Autodesk Fusion 360 part; units mm, degrees
note: some values were not read from the file. Set by a fixed rule: which sketch regions a step uses.
(part 43 of 59)
  spline S54 degree 5 poles (24.6806, -2.8132) (24.6807, -2.8132) (24.6809, -2.8133) (24.6812, -2.8135) (24.6816, -2.8138) (24.6822, -2.8142) (24.683, -2.8146) (24.6838, -2.8151) (24.6848, -2.8157) (24.6858, -2.8163) (24.6869, -2.8169) (24.6881, -2.8177) (24.6895, -2.8184) (24.6909, -2.8193) (24.6924, -2.8201) (24.694, -2.821) (24.6956, -2.822) (24.6974, -2.823) (24.6993, -2.8241) (24.7012, -2.8252) (24.7033, -2.8263) (24.7054, -2.8275) (24.7076, -2.8287) (24.7099, -2.83) (24.7122, -2.8313) (24.7147, -2.8327) (24.7172, -2.8341) (24.7198, -2.8355) (24.7225, -2.837) (24.7253, -2.8385) (24.7282, -2.84) (24.7311, -2.8416) (24.7341, -2.8432) (24.7372, -2.8449) (24.7404, -2.8465) (24.7437, -2.8482) (24.747, -2.85) (24.7504, -2.8518) (24.7539, -2.8536) (24.7574, -2.8554) (24.761, -2.8573) (24.7647, -2.8592) (24.7685, -2.8611) (24.7723, -2.8631) (24.7763, -2.8651) (24.7802, -2.8671) (24.7843, -2.8691) (24.7884, -2.8712) (24.7926, -2.8733) (24.7969, -2.8754) (24.8012, -2.8775) (24.8056, -2.8797) (24.8101, -2.8819) (24.8147, -2.8841) (24.8193, -2.8863) (24.8239, -2.8886) (24.8287, -2.8909) (24.8335, -2.8932) (24.8384, -2.8955) (24.8433, -2.8979) (24.8483, -2.9002) (24.8534, -2.9026) (24.8585, -2.905) (24.8637, -2.9075) (24.869, -2.9099) (24.8743, -2.9124) (24.8797, -2.9149) (24.8852, -2.9174) (24.8907, -2.9199) (24.8962, -2.9224) (24.9019, -2.925) (24.9076, -2.9275) (24.9133, -2.9301) (24.9192, -2.9327) (24.925, -2.9353) (24.931, -2.938) (24.937, -2.9406) (24.943, -2.9433) (24.9492, -2.946) (24.9553, -2.9486) (24.9616, -2.9514) (24.9679, -2.9541) (24.9742, -2.9568) (24.9806, -2.9595) (24.9871, -2.9623) (24.9936, -2.9651) (25.0002, -2.9678) (25.0069, -2.9706) (25.0136, -2.9734) (25.0203, -2.9762) (25.0271, -2.9791) (25.034, -2.9819) (25.0409, -2.9848) (25.0479, -2.9876) (25.0549, -2.9905) (25.062, -2.9933) (25.0691, -2.9962) (25.0763, -2.9991) (25.0836, -3.002) (25.0909, -3.0049) (25.0982, -3.0078) (25.1056, -3.0108) (25.1131, -3.0137) (25.1206, -3.0166) (25.1282, -3.0196) (25.1358, -3.0226) (25.1434, -3.0255) (25.1512, -3.0285) (25.1589, -3.0315) (25.1668, -3.0344) (25.1746, -3.0374) (25.1826, -3.0404) (25.1905, -3.0434) (25.1986, -3.0464) (25.2066, -3.0494) (25.2148, -3.0524) (25.2229, -3.0555) (25.2312, -3.0585) (25.2394, -3.0615) (25.2478, -3.0645) (25.2562, -3.0676) (25.2646, -3.0706) (25.2731, -3.0737) (25.2816, -3.0767) (25.2901, -3.0798) (25.2988, -3.0828) (25.3074, -3.0859) (25.3161, -3.0889) (25.3249, -3.092) (25.3337, -3.095) (25.3426, -3.0981) (25.3515, -3.1012) (25.3604, -3.1042) (25.3694, -3.1073) (25.3785, -3.1104) (25.3876, -3.1134) (25.3967, -3.1165) (25.4059, -3.1196) (25.4151, -3.1227) (25.4244, -3.1257) (25.4337, -3.1288) (25.4431, -3.1319) (25.4525, -3.135) (25.462, -3.138) (25.4715, -3.1411) (25.481, -3.1442) (25.4906, -3.1473) (25.5003, -3.1503) (25.5099, -3.1534) (25.5197, -3.1565) (25.5294, -3.1596) (25.5393, -3.1626) (25.5491, -3.1657) (25.559, -3.1688) (25.569, -3.1718) (25.579, -3.1749) (25.589, -3.1779) (25.5991, -3.181) (25.6092, -3.1841) (25.6194, -3.1871) (25.6296, -3.1902) (25.6398, -3.1932) (25.6501, -3.1963) (25.6604, -3.1993) (25.6708, -3.2023) (25.6812, -3.2054) (25.6917, -3.2084) (25.7022, -3.2114) (25.7127, -3.2145) (25.7233, -3.2175) (25.7339, -3.2205) (25.7446, -3.2235) (25.7553, -3.2265) (25.766, -3.2295) (25.7768, -3.2325) (25.7877, -3.2355) (25.7985, -3.2385) (25.8094, -3.2415) (25.8204, -3.2445) (25.8314, -3.2475) (25.8424, -3.2504) (25.8535, -3.2534) (25.8646, -3.2564) (25.8757, -3.2593) (25.8869, -3.2623) (25.8982, -3.2652) (25.9094, -3.2682) (25.9207, -3.2711) (25.9321, -3.274) (25.9435, -3.2769) (25.9549, -3.2798) (25.9663, -3.2828) (25.9778, -3.2857) (25.9894, -3.2886) (26.001, -3.2914) (26.0126, -3.2943) (26.0242, -3.2972) (26.0359, -3.3001) (26.0477, -3.3029) (26.0594, -3.3058) (26.0712, -3.3086) (26.0831, -3.3115) (26.095, -3.3143) (26.1069, -3.3171) (26.1188, -3.3199) (26.1308, -3.3227) (26.1428, -3.3255) (26.1549, -3.3283) (26.167, -3.3311) (26.1792, -3.3339) (26.1913, -3.3367) (26.2035, -3.3394) (26.2158, -3.3422) (26.2281, -3.3449) (26.2404, -3.3477) (26.2528, -3.3504) (26.2651, -3.3531) (26.2776, -3.3558) (26.29, -3.3585) (26.3025, -3.3612) (26.3151, -3.3639) (26.3276, -3.3666) (26.3403, -3.3692) (26.3529, -3.3719) (26.3656, -3.3745) (26.3783, -3.3771) (26.391, -3.3798) (26.4038, -3.3824) (26.4166, -3.385) (26.4295, -3.3876) (26.4424, -3.3902) (26.4553, -3.3927) (26.4682, -3.3953) (26.4812, -3.3979) (26.4943, -3.4004) (26.5073, -3.4029) (26.5204, -3.4055) (26.5335, -3.408) (26.5467, -3.4105) (26.5599, -3.413) (26.5731, -3.4154) (26.5837, -3.4174) (26.5917, -3.4189) (26.597, -3.4199) (26.5997, -3.4204) knots 0 0 0 0 0 0 0.00416667 0.00833333 0.0125 0.01666667 0.02083333 0.025 0.02916667 0.03333333 0.0375 0.04166667 0.04583333 0.05 0.05416667 0.05833333 0.0625 0.06666667 0.07083333 0.075 0.07916667 0.08333333 0.0875 0.09166667 0.09583333 0.1 0.10416667 0.10833333 0.1125 0.11666667 0.12083333 0.125 0.12916667 0.13333333 0.1375 0.14166667 0.14583333 0.15 0.15416667 0.15833333 0.1625 0.16666667 0.17083333 0.175 0.17916667 0.18333333 0.1875 0.19166667 0.19583333 0.2 0.20416667 0.20833333 0.2125 0.21666667 0.22083333 0.225 0.22916667 0.23333333 0.2375 0.24166667 0.24583333 0.25 0.25416667 0.25833333 0.2625 0.26666667 0.27083333 0.275 0.27916667 0.28333333 0.2875 0.29166667 0.29583333 0.3 0.30416667 0.30833333 0.3125 0.31666667 0.32083333 0.325 0.32916667 0.33333333 0.3375 0.34166667 0.34583333 0.35 0.35416667 0.35833333 0.3625 0.36666667 0.37083333 0.375 0.37916667 0.38333333 0.3875 0.39166667 0.39583333 0.4 0.40416667 0.40833333 0.4125 0.41666667 0.42083333 0.425 0.42916667 0.43333333 0.4375 0.44166667 0.44583333 0.45 0.45416667 0.45833333 0.4625 0.46666667 0.47083333 0.475 0.47916667 0.48333333 0.4875 0.49166667 0.49583333 0.5 0.50416667 0.50833333 0.5125 0.51666667 0.52083333 0.525 0.52916667 0.53333333 0.5375 0.54166667 0.54583333 0.55 0.55416667 0.55833333 0.5625 0.56666667 0.57083333 0.575 0.57916667 0.58333333 0.5875 0.59166667 0.59583333 0.6 0.60416667 0.60833333 0.6125 0.61666667 0.62083333 0.625 0.62916667 0.63333333 0.6375 0.64166667 0.64583333 0.65 0.65416667 0.65833333 0.6625 0.66666667 0.67083333 0.675 0.67916667 0.68333333 0.6875 0.69166667 0.69583333 0.7 0.70416667 0.70833333 0.7125 0.71666667 0.72083333 0.725 0.72916667 0.73333333 0.7375 0.74166667 0.74583333 0.75 0.75416667 0.75833333 0.7625 0.76666667 0.77083333 0.775 0.77916667 0.78333333 0.7875 0.79166667 0.79583333 0.8 0.80416667 0.80833333 0.8125 0.81666667 0.82083333 0.825 0.82916667 0.83333333 0.8375 0.84166667 0.84583333 0.85 0.85416667 0.85833333 0.8625 0.86666667 0.87083333 0.875 0.87916667 0.88333333 0.8875 0.89166667 0.89583333 0.9 0.90416667 0.90833333 0.9125 0.91666667 0.92083333 0.925 0.92916667 0.93333333 0.9375 0.94166667 0.94583333 0.95 0.95416667 0.95833333 0.9625 0.96666667 0.97083333 0.975 0.97916667 0.98333333 0.9875 0.99166667 0.99583333 1 1 1 1 1 1
  arc A55 (26.5997, -3.4204) -> (27.0873, -2.5758) centre (0, 12.5) ccw
  spline S55 degree 5 poles (27.0873, -2.5758) (27.0855, -2.5737) (27.082, -2.5696) (27.0767, -2.5635) (27.0697, -2.5553) (27.061, -2.545) (27.0522, -2.5349) (27.0435, -2.5247) (27.0347, -2.5146) (27.026, -2.5045) (27.0173, -2.4945) (27.0086, -2.4845) (26.9999, -2.4745) (26.9912, -2.4646) (26.9825, -2.4547) (26.9738, -2.4448) (26.9651, -2.435) (26.9565, -2.4252) (26.9478, -2.4154) (26.9392, -2.4057) (26.9305, -2.396) (26.9219, -2.3863) (26.9133, -2.3767) (26.9047, -2.3671) (26.8961, -2.3576) (26.8875, -2.3481) (26.8789, -2.3386) (26.8703, -2.3291) (26.8618, -2.3197) (26.8532, -2.3104) (26.8447, -2.301) (26.8361, -2.2917) (26.8276, -2.2824) (26.8191, -2.2732) (26.8106, -2.264) (26.8021, -2.2549) (26.7937, -2.2457) (26.7852, -2.2366) (26.7767, -2.2276) (26.7683, -2.2186) (26.7599, -2.2096) (26.7515, -2.2006) (26.7431, -2.1917) (26.7347, -2.1829) (26.7263, -2.174) (26.7179, -2.1652) (26.7096, -2.1565) (26.7012, -2.1477) (26.6929, -2.139) (26.6846, -2.1304) (26.6763, -2.1218) (26.668, -2.1132) (26.6597, -2.1046) (26.6514, -2.0961) (26.6432, -2.0877) (26.635, -2.0792) (26.6267, -2.0708) (26.6185, -2.0625) (26.6103, -2.0541) (26.6022, -2.0459) (26.594, -2.0376) (26.5858, -2.0294) (26.5777, -2.0212) (26.5696, -2.0131) (26.5615, -2.005) (26.5534, -1.9969) (26.5453, -1.9889) (26.5373, -1.9809) (26.5292, -1.9729) (26.5212, -1.965) (26.5132, -1.9571) (26.5052, -1.9493) (26.4972, -1.9415) (26.4893, -1.9337) (26.4813, -1.926) (26.4734, -1.9183) (26.4655, -1.9106) (26.4576, -1.903) (26.4497, -1.8954) (26.4419, -1.8879) (26.434, -1.8804) (26.4262, -1.8729) (26.4184, -1.8655) (26.4106, -1.8581) (26.4029, -1.8508) (26.3951, -1.8435) (26.3874, -1.8362) (26.3797, -1.8289) (26.372, -1.8217) (26.3643, -1.8146) (26.3567, -1.8075) (26.3491, -1.8004) (26.3414, -1.7933) (26.3339, -1.7863) (26.3263, -1.7794) (26.3188, -1.7724) (26.3112, -1.7656) (26.3037, -1.7587) (26.2962, -1.7519) (26.2888, -1.7451) (26.2813, -1.7384) (26.2739, -1.7317) (26.2665, -1.725) (26.2592, -1.7184) (26.2518, -1.7119) (26.2445, -1.7053) (26.2372, -1.6988) (26.2299, -1.6924) (26.2227, -1.6859) (26.2154, -1.6796) (26.2082, -1.6732) (26.201, -1.6669) (26.1939, -1.6607) (26.1868, -1.6544) (26.1796, -1.6483) (26.1726, -1.6421) (26.1655, -1.636) (26.1585, -1.63) (26.1515, -1.6239) (26.1445, -1.618) (26.1375, -1.612) (26.1306, -1.6061) (26.1237, -1.6003) (26.1168, -1.5945) (26.11, -1.5887) (26.1032, -1.5829) (26.0964, -1.5772) (26.0896, -1.5716) (26.0829, -1.566) (26.0762, -1.5604) (26.0695, -1.5549) (26.0629, -1.5494) (26.0563, -1.5439) (26.0497, -1.5385) (26.0431, -1.5332) (26.0366, -1.5278) (26.0301, -1.5225) (26.0236, -1.5173) (26.0172, -1.5121) (26.0108, -1.5069) (26.0044, -1.5018) (25.9981, -1.4967) (25.9918, -1.4917) (25.9855, -1.4867) (25.9793, -1.4818) (25.9731, -1.4769) (25.9669, -1.472) (25.9608, -1.4672) (25.9547, -1.4624) (25.9486, -1.4576) (25.9426, -1.4529) (25.9366, -1.4483) (25.9306, -1.4437) (25.9247, -1.4391) (25.9188, -1.4346) (25.913, -1.4301) (25.9072, -1.4257) (25.9014, -1.4213) (25.8957, -1.4169) (25.89, -1.4126) (25.8843, -1.4083) (25.8787, -1.4041) (25.8731, -1.3999) (25.8676, -1.3958) (25.8621, -1.3917) (25.8566, -1.3876) (25.8512, -1.3836) (25.8458, -1.3797) (25.8405, -1.3758) (25.8352, -1.3719) (25.8299, -1.3681) (25.8247, -1.3643) (25.8195, -1.3605) (25.8144, -1.3568) (25.8093, -1.3532) (25.8043, -1.3496) (25.7993, -1.346) (25.7944, -1.3425) (25.7895, -1.339) (25.7847, -1.3356) (25.7799, -1.3322) (25.7751, -1.3289) (25.7704, -1.3256) (25.7658, -1.3224) (25.7612, -1.3192) (25.7566, -1.316) (25.7521, -1.3129) (25.7476, -1.3098) (25.7432, -1.3068) (25.7389, -1.3039) (25.7346, -1.3009) (25.7304, -1.2981) (25.7262, -1.2952) (25.722, -1.2925) (25.718, -1.2897) (25.7139, -1.287) (25.71, -1.2844) (25.706, -1.2818) (25.7022, -1.2793) (25.6984, -1.2768) (25.6947, -1.2743) (25.691, -1.2719) (25.6874, -1.2696) (25.6838, -1.2673) (25.6803, -1.265) (25.6769, -1.2628) (25.6735, -1.2607) (25.6702, -1.2586) (25.667, -1.2565) (25.6638, -1.2545) (25.6607, -1.2526) (25.6577, -1.2506) (25.6547, -1.2488) (25.6518, -1.247) (25.6489, -1.2452) (25.6462, -1.2435) (25.6435, -1.2419) (25.6409, -1.2403) (25.6383, -1.2387) (25.6358, -1.2372) (25.6334, -1.2358) (25.6311, -1.2344) (25.6289, -1.233) (25.6267, -1.2317) (25.6246, -1.2305) (25.6226, -1.2293) (25.6207, -1.2282) (25.6188, -1.2271) (25.6171, -1.2261) (25.6154, -1.2251) (25.6138, -1.2242) (25.6123, -1.2233) (25.6109, -1.2225) (25.6096, -1.2217) (25.6083, -1.221) (25.6072, -1.2204) (25.6061, -1.2198) (25.6052, -1.2193) (25.6043, -1.2188) (25.6036, -1.2184) (25.6029, -1.218) (25.6025, -1.2178) (25.6022, -1.2176) (25.602, -1.2175) (25.6019, -1.2175) knots -1 -1 -1 -1 -1 -1 -0.99583333 -0.99166667 -0.9875 -0.98333333 -0.97916667 -0.975 -0.97083333 -0.96666667 -0.9625 -0.95833333 -0.95416667 -0.95 -0.94583333 -0.94166667 -0.9375 -0.93333333 -0.92916667 -0.925 -0.92083333 -0.91666667 -0.9125 -0.90833333 -0.90416667 -0.9 -0.89583333 -0.89166667 -0.8875 -0.88333333 -0.87916667 -0.875 -0.87083333 -0.86666667 -0.8625 -0.85833333 -0.85416667 -0.85 -0.84583333 -0.84166667 -0.8375 -0.83333333 -0.82916667 -0.825 -0.82083333 -0.81666667 -0.8125 -0.80833333 -0.80416667 -0.8 -0.79583333 -0.79166667 -0.7875 -0.78333333 -0.77916667 -0.775 -0.77083333 -0.76666667 -0.7625 -0.75833333 -0.75416667 -0.75 -0.74583333 -0.74166667 -0.7375 -0.73333333 -0.72916667 -0.725 -0.72083333 -0.71666667 -0.7125 -0.70833333 -0.70416667 -0.7 -0.69583333 -0.69166667 -0.6875 -0.68333333 -0.67916667 -0.675 -0.67083333 -0.66666667 -0.6625 -0.65833333 -0.65416667 -0.65 -0.64583333 -0.64166667 -0.6375 -0.63333333 -0.62916667 -0.625 -0.62083333 -0.61666667 -0.6125 -0.60833333 -0.60416667 -0.6 -0.59583333 -0.59166667 -0.5875 -0.58333333 -0.57916667 -0.575 -0.57083333 -0.56666667 -0.5625 -0.55833333 -0.55416667 -0.55 -0.54583333 -0.54166667 -0.5375 -0.53333333 -0.52916667 -0.525 -0.52083333 -0.51666667 -0.5125 -0.50833333 -0.50416667 -0.5 -0.49583333 -0.49166667 -0.4875 -0.48333333 -0.47916667 -0.475 -0.47083333 -0.46666667 -0.4625 -0.45833333 -0.45416667 -0.45 -0.44583333 -0.44166667 -0.4375 -0.43333333 -0.42916667 -0.425 -0.42083333 -0.41666667 -0.4125 -0.40833333 -0.40416667 -0.4 -0.39583333 -0.39166667 -0.3875 -0.38333333 -0.37916667 -0.375 -0.37083333 -0.36666667 -0.3625 -0.35833333 -0.35416667 -0.35 -0.34583333 -0.34166667 -0.3375 -0.33333333 -0.32916667 -0.325 -0.32083333 -0.31666667 -0.3125 -0.30833333 -0.30416667 -0.3 -0.29583333 -0.29166667 -0.2875 -0.28333333 -0.27916667 -0.275 -0.27083333 -0.26666667 -0.2625 -0.25833333 -0.25416667 -0.25 -0.24583333 -0.24166667 -0.2375 -0.23333333 -0.22916667 -0.225 -0.22083333 -0.21666667 -0.2125 -0.20833333 -0.20416667 -0.2 -0.19583333 -0.19166667 -0.1875 -0.18333333 -0.17916667 -0.175 -0.17083333 -0.16666667 -0.1625 -0.15833333 -0.15416667 -0.15 -0.14583333 -0.14166667 -0.1375 -0.13333333 -0.12916667 -0.125 -0.12083333 -0.11666667 -0.1125 -0.10833333 -0.10416667 -0.1 -0.09583333 -0.09166667 -0.0875 -0.08333333 -0.07916667 -0.075 -0.07083333 -0.06666667 -0.0625 -0.05833333 -0.05416667 -0.05 -0.04583333 -0.04166667 -0.0375 -0.03333333 -0.02916667 -0.025 -0.02083333 -0.01666667 -0.0125 -0.00833333 -0.00416667 0 0 0 0 0 0
  line L119 (25.6019, -1.2175) -> (25.6012, -1.2171)
  line L120 (25.6012, -1.2171) -> (25.3417, -1.078)
  arc A56 (25.3417, -1.078) -> (25.8803, -0.0209) centre (0, 12.5) ccw
  line L121 (25.8803, -0.0209) -> (26.1453, -0.1491)
  line L122 (26.1453, -0.1491) -> (26.1461, -0.1495)
  spline S56 degree 5 poles (26.1461, -0.1495) (26.1462, -0.1495) (26.1464, -0.1496) (26.1467, -0.1497) (26.1471, -0.15) (26.1478, -0.1503) (26.1486, -0.1506) (26.1495, -0.151) (26.1504, -0.1515) (26.1515, -0.152) (26.1527, -0.1526) (26.154, -0.1531) (26.1554, -0.1538) (26.1569, -0.1544) (26.1585, -0.1551) (26.1602, -0.1559) (26.1619, -0.1567) (26.1638, -0.1575) (26.1658, -0.1583) (26.1678, -0.1592) (26.17, -0.1602) (26.1722, -0.1611) (26.1745, -0.1621) (26.1769, -0.1631) (26.1794, -0.1642) (26.182, -0.1653) (26.1847, -0.1664) (26.1874, -0.1676) (26.1903, -0.1687) (26.1932, -0.1699) (26.1962, -0.1712) (26.1993, -0.1724) (26.2024, -0.1737) (26.2057, -0.175) (26.209, -0.1764) (26.2124, -0.1778) (26.2159, -0.1791) (26.2195, -0.1806) (26.2231, -0.182) (26.2269, -0.1834) (26.2307, -0.1849) (26.2345, -0.1864) (26.2385, -0.188) (26.2425, -0.1895) (26.2466, -0.1911) (26.2508, -0.1927) (26.255, -0.1943) (26.2594, -0.1959) (26.2638, -0.1975) (26.2682, -0.1992) (26.2728, -0.2009) (26.2774, -0.2026) (26.282, -0.2043) (26.2868, -0.206) (26.2916, -0.2077) (26.2965, -0.2095) (26.3015, -0.2113) (26.3065, -0.2131) (26.3116, -0.2149) (26.3167, -0.2167) (26.322, -0.2185) (26.3273, -0.2204) (26.3326, -0.2222) (26.338, -0.2241) (26.3435, -0.226) (26.3491, -0.2279) (26.3547, -0.2298) (26.3604, -0.2317) (26.3661, -0.2336) (26.3719, -0.2356) (26.3778, -0.2375) (26.3837, -0.2395) (26.3897, -0.2414) (26.3958, -0.2434) (26.4019, -0.2454) (26.4081, -0.2474) (26.4144, -0.2494) (26.4207, -0.2514) (26.427, -0.2534) (26.4335, -0.2555) (26.4399, -0.2575) (26.4465, -0.2596) (26.4531, -0.2616) (26.4598, -0.2637) (26.4665, -0.2657) (26.4733, -0.2678) (26.4801, -0.2699) (26.487, -0.272) (26.4939, -0.274) (26.5009, -0.2761) (26.508, -0.2782) (26.5151, -0.2803) (26.5223, -0.2824) (26.5296, -0.2845) (26.5368, -0.2867) (26.5442, -0.2888) (26.5516, -0.2909) (26.559, -0.293) (26.5665, -0.2952) (26.5741, -0.2973) (26.5817, -0.2994) (26.5894, -0.3016) (26.5971, -0.3037) (26.6049, -0.3058) (26.6127, -0.308) (26.6206, -0.3101) (26.6286, -0.3123) (26.6365, -0.3144) (26.6446, -0.3166) (26.6527, -0.3187) (26.6608, -0.3208) (26.669, -0.323) (26.6773, -0.3251) (26.6856, -0.3273) (26.6939, -0.3294) (26.7023, -0.3316) (26.7108, -0.3337) (26.7193, -0.3359) (26.7278, -0.338) (26.7364, -0.3402) (26.7451, -0.3423) (26.7537, -0.3445) (26.7625, -0.3466) (26.7713, -0.3487) (26.7801, -0.3509) (26.789, -0.353) (26.798, -0.3551) (26.8069, -0.3573) (26.816, -0.3594) (26.8251, -0.3615) (26.8342, -0.3636) (26.8434, -0.3658) (26.8526, -0.3679) (26.8619, -0.37) (26.8712, -0.3721) (26.8806, -0.3742) (26.89, -0.3763) (26.8994, -0.3784) (26.9089, -0.3805) (26.9185, -0.3826) (26.9281, -0.3847) (26.9377, -0.3867) (26.9474, -0.3888) (26.9571, -0.3909) (26.9669, -0.3929) (26.9767, -0.395) (26.9866, -0.3971) (26.9965, -0.3991) (27.0064, -0.4011) (27.0164, -0.4032) (27.0265, -0.4052) (27.0365, -0.4072) (27.0467, -0.4093) (27.0568, -0.4113) (27.0671, -0.4133) (27.0773, -0.4153) (27.0876, -0.4173) (27.0979, -0.4193) (27.1083, -0.4213) (27.1188, -0.4232) (27.1292, -0.4252) (27.1397, -0.4272) (27.1503, -0.4291) (27.1609, -0.4311) (27.1715, -0.433) (27.1822, -0.4349) (27.1929, -0.4368) (27.2037, -0.4388) (27.2145, -0.4407) (27.2253, -0.4426) (27.2362, -0.4445) (27.2471, -0.4463) (27.2581, -0.4482) (27.2691, -0.4501) (27.2801, -0.4519) (27.2912, -0.4538) (27.3023, -0.4556) (27.3135, -0.4574) (27.3247, -0.4593) (27.3359, -0.4611) (27.3472, -0.4629) (27.3585, -0.4647) (27.3699, -0.4665) (27.3813, -0.4682) (27.3927, -0.47) (27.4042, -0.4718) (27.4157, -0.4735) (27.4273, -0.4752) (27.4388, -0.477) (27.4505, -0.4787) (27.4621, -0.4804) (27.4738, -0.4821) (27.4856, -0.4838) (27.4974, -0.4854) (27.5092, -0.4871) (27.521, -0.4887) (27.5329, -0.4904) (27.5449, -0.492) (27.5568, -0.4936) (27.5688, -0.4952) (27.5809, -0.4968) (27.5929, -0.4984) (27.605, -0.5) (27.6172, -0.5016) (27.6294, -0.5031) (27.6416, -0.5047) (27.6539, -0.5062) (27.6661, -0.5077) (27.6785, -0.5092) (27.6908, -0.5107) (27.7032, -0.5122) (27.7157, -0.5136) (27.7281, -0.5151) (27.7406, -0.5165) (27.7532, -0.518) (27.7658, -0.5194) (27.7784, -0.5208) (27.791, -0.5222) (27.8037, -0.5236) (27.8164, -0.5249) (27.8291, -0.5263) (27.8419, -0.5276) (27.8547, -0.529) (27.8676, -0.5303) (27.8805, -0.5316) (27.8934, -0.5329) (27.9063, -0.5342) (27.9193, -0.5354) (27.9323, -0.5367) (27.9454, -0.5379) (27.9585, -0.5391) (27.9716, -0.5404) (27.9848, -0.5415) (27.9979, -0.5427) (28.0112, -0.5439) (28.0244, -0.5451) (28.0377, -0.5462) (28.051, -0.5473) (28.0644, -0.5484) (28.0777, -0.5495) (28.0911, -0.5506) (28.1019, -0.5515) (28.11, -0.5521) (28.1154, -0.5525) (28.1181, -0.5527) knots 0 0 0 0 0 0 0.00416667 0.00833333 0.0125 0.01666667 0.02083333 0.025 0.02916667 0.03333333 0.0375 0.04166667 0.04583333 0.05 0.05416667 0.05833333 0.0625 0.06666667 0.07083333 0.075 0.07916667 0.08333333 0.0875 0.09166667 0.09583333 0.1 0.10416667 0.10833333 0.1125 0.11666667 0.12083333 0.125 0.12916667 0.13333333 0.1375 0.14166667 0.14583333 0.15 0.15416667 0.15833333 0.1625 0.16666667 0.17083333 0.175 0.17916667 0.18333333 0.1875 0.19166667 0.19583333 0.2 0.20416667 0.20833333 0.2125 0.21666667 0.22083333 0.225 0.22916667 0.23333333 0.2375 0.24166667 0.24583333 0.25 0.25416667 0.25833333 0.2625 0.26666667 0.27083333 0.275 0.27916667 0.28333333 0.2875 0.29166667 0.29583333 0.3 0.30416667 0.30833333 0.3125 0.31666667 0.32083333 0.325 0.32916667 0.33333333 0.3375 0.34166667 0.34583333 0.35 0.35416667 0.35833333 0.3625 0.36666667 0.37083333 0.375 0.37916667 0.38333333 0.3875 0.39166667 0.39583333 0.4 0.40416667 0.40833333 0.4125 0.41666667 0.42083333 0.425 0.42916667 0.43333333 0.4375 0.44166667 0.44583333 0.45 0.45416667 0.45833333 0.4625 0.46666667 0.47083333 0.475 0.47916667 0.48333333 0.4875 0.49166667 0.49583333 0.5 0.50416667 0.50833333 0.5125 0.51666667 0.52083333 0.525 0.52916667 0.53333333 0.5375 0.54166667 0.54583333 0.55 0.55416667 0.55833333 0.5625 0.56666667 0.57083333 0.575 0.57916667 0.58333333 0.5875 0.59166667 0.59583333 0.6 0.60416667 0.60833333 0.6125 0.61666667 0.62083333 0.625 0.62916667 0.63333333 0.6375 0.64166667 0.64583333 0.65 0.65416667 0.65833333 0.6625 0.66666667 0.67083333 0.675 0.67916667 0.68333333 0.6875 0.69166667 0.69583333 0.7 0.70416667 0.70833333 0.7125 0.71666667 0.72083333 0.725 0.72916667 0.73333333 0.7375 0.74166667 0.74583333 0.75 0.75416667 0.75833333 0.7625 0.76666667 0.77083333 0.775 0.77916667 0.78333333 0.7875 0.79166667 0.79583333 0.8 0.80416667 0.80833333 0.8125 0.81666667 0.82083333 0.825 0.82916667 0.83333333 0.8375 0.84166667 0.84583333 0.85 0.85416667 0.85833333 0.8625 0.86666667 0.87083333 0.875 0.87916667 0.88333333 0.8875 0.89166667 0.89583333 0.9 0.90416667 0.90833333 0.9125 0.91666667 0.92083333 0.925 0.92916667 0.93333333 0.9375 0.94166667 0.94583333 0.95 0.95416667 0.95833333 0.9625 0.96666667 0.97083333 0.975 0.97916667 0.98333333 0.9875 0.99166667 0.99583333 1 1 1 1 1 1
  arc A57 (28.1181, -0.5527) -> (28.5147, 0.3382) centre (0, 12.5) ccw
  spline S57 degree 5 poles (28.5147, 0.3382) (28.5128, 0.34) (28.5089, 0.3438) (28.503, 0.3494) (28.4951, 0.3568) (28.4854, 0.366) (28.4756, 0.3752) (28.4658, 0.3844) (28.4561, 0.3935) (28.4464, 0.4027) (28.4366, 0.4117) (28.4269, 0.4208) (28.4172, 0.4298) (28.4075, 0.4387) (28.3978, 0.4477) (28.3882, 0.4566) (28.3785, 0.4655) (28.3689, 0.4743) (28.3593, 0.4831) (28.3496, 0.4919) (28.34, 0.5006) (28.3305, 0.5093) (28.3209, 0.518) (28.3113, 0.5266) (28.3018, 0.5352) (28.2922, 0.5438) (28.2827, 0.5523) (28.2732, 0.5608) (28.2637, 0.5693) (28.2542, 0.5777) (28.2447, 0.5861) (28.2353, 0.5945) (28.2259, 0.6028) (28.2164, 0.6111) (28.207, 0.6193) (28.1976, 0.6276) (28.1882, 0.6357) (28.1789, 0.6439) (28.1695, 0.652) (28.1602, 0.6601) (28.1509, 0.6682) (28.1416, 0.6762) (28.1323, 0.6842) (28.123, 0.6921) (28.1137, 0.7) (28.1045, 0.7079) (28.0953, 0.7157) (28.0861, 0.7235) (28.0769, 0.7313) (28.0677, 0.7391) (28.0585, 0.7468) (28.0494, 0.7544) (28.0403, 0.7621) (28.0312, 0.7697) (28.0221, 0.7772) (28.013, 0.7847) (28.0039, 0.7922) (27.9949, 0.7997) (27.9859, 0.8071) (27.9769, 0.8145) (27.9679, 0.8219) (27.9589, 0.8292) (27.95, 0.8365) (27.9411, 0.8437) (27.9322, 0.8509) (27.9233, 0.8581) (27.9144, 0.8652) (27.9055, 0.8724) (27.8967, 0.8794) (27.8879, 0.8865) (27.8791, 0.8935) (27.8704, 0.9004) (27.8616, 0.9073) (27.8529, 0.9142) (27.8442, 0.9211) (27.8355, 0.9279) (27.8268, 0.9347) (27.8182, 0.9415) (27.8096, 0.9482) (27.801, 0.9548) (27.7924, 0.9615) (27.7838, 0.9681) (27.7753, 0.9747) (27.7668, 0.9812) (27.7583, 0.9877) (27.7498, 0.9942) (27.7414, 1.0006) (27.733, 1.007) (27.7246, 1.0133) (27.7162, 1.0197) (27.7078, 1.0259) (27.6995, 1.0322) (27.6912, 1.0384) (27.6829, 1.0446) (27.6747, 1.0507) (27.6665, 1.0568) (27.6582, 1.0629) (27.6501, 1.0689) (27.6419, 1.0749) (27.6338, 1.0808) (27.6257, 1.0868) (27.6176, 1.0926) (27.6096, 1.0985) (27.6015, 1.1043) (27.5936, 1.1101) (27.5856, 1.1158) (27.5776, 1.1215) (27.5697, 1.1272) (27.5618, 1.1328) (27.554, 1.1384) (27.5462, 1.1439) (27.5384, 1.1494) (27.5306, 1.1549) (27.5228, 1.1604) (27.5151, 1.1658) (27.5074, 1.1711) (27.4998, 1.1765) (27.4922, 1.1817) (27.4846, 1.187) (27.477, 1.1922) (27.4695, 1.1974) (27.462, 1.2025) (27.4545, 1.2076) (27.447, 1.2127) (27.4396, 1.2177) (27.4323, 1.2227) (27.4249, 1.2277) (27.4176, 1.2326) (27.4103, 1.2375) (27.4031, 1.2423) (27.3958, 1.2471) (27.3887, 1.2519) (27.3815, 1.2566) (27.3744, 1.2613) (27.3673, 1.266) (27.3603, 1.2706) (27.3533, 1.2752) (27.3463, 1.2797) (27.3393, 1.2842) (27.3324, 1.2887) (27.3256, 1.2931) (27.3187, 1.2975) (27.3119, 1.3018) (27.3052, 1.3061) (27.2985, 1.3104) (27.2918, 1.3146) (27.2851, 1.3188) (27.2785, 1.323) (27.272, 1.3271) (27.2654, 1.3312) (27.259, 1.3352) (27.2525, 1.3392) (27.2461, 1.3432) (27.2397, 1.3471) (27.2334, 1.351) (27.2271, 1.3549) (27.2209, 1.3587) (27.2147, 1.3624) (27.2085, 1.3662) (27.2024, 1.3699) (27.1963, 1.3735) (27.1903, 1.3771) (27.1843, 1.3807) (27.1784, 1.3842) (27.1725, 1.3877) (27.1666, 1.3912) (27.1608, 1.3946) (27.155, 1.398) (27.1493, 1.4013) (27.1436, 1.4046) (27.138, 1.4079) (27.1324, 1.4111) (27.1269, 1.4143) (27.1214, 1.4174) (27.116, 1.4205) (27.1106, 1.4236) (27.1053, 1.4266) (27.1, 1.4296) (27.0948, 1.4325) (27.0896, 1.4354) (27.0845, 1.4383) (27.0794, 1.4411) (27.0744, 1.4439) (27.0694, 1.4466) (27.0645, 1.4493) (27.0597, 1.452) (27.0549, 1.4546) (27.0501, 1.4572) (27.0454, 1.4597) (27.0408, 1.4622) (27.0362, 1.4647) (27.0317, 1.4671) (27.0272, 1.4694) (27.0228, 1.4718) (27.0185, 1.4741) (27.0142, 1.4763) (27.01, 1.4785) (27.0058, 1.4807) (27.0017, 1.4828) (26.9977, 1.4849) (26.9937, 1.4869) (26.9898, 1.4889) (26.986, 1.4909) (26.9822, 1.4928) (26.9785, 1.4947) (26.9748, 1.4965) (26.9713, 1.4983) (26.9678, 1.5001) (26.9643, 1.5018) (26.961, 1.5034) (26.9577, 1.5051) (26.9544, 1.5066) (26.9513, 1.5082) (26.9482, 1.5097) (26.9452, 1.5111) (26.9423, 1.5125) (26.9394, 1.5139) (26.9366, 1.5152) (26.9339, 1.5165) (26.9313, 1.5177) (26.9288, 1.5189) (26.9263, 1.5201) (26.924, 1.5212) (26.9217, 1.5222) (26.9195, 1.5232) (26.9173, 1.5242) (26.9153, 1.5251) (26.9134, 1.526) (26.9115, 1.5269) (26.9097, 1.5276) (26.908, 1.5284) (26.9065, 1.5291) (26.905, 1.5298) (26.9036, 1.5304) (26.9023, 1.5309) (26.9011, 1.5315) (26.9, 1.5319) (26.899, 1.5324) (26.8981, 1.5328) (26.8973, 1.5331) (26.8966, 1.5334) (26.8961, 1.5336) (26.8958, 1.5337) (26.8956, 1.5338) (26.8955, 1.5338) knots -1 -1 -1 -1 -1 -1 -0.99583333 -0.99166667 -0.9875 -0.98333333 -0.97916667 -0.975 -0.97083333 -0.96666667 -0.9625 -0.95833333 -0.95416667 -0.95 -0.94583333 -0.94166667 -0.9375 -0.93333333 -0.92916667 -0.925 -0.92083333 -0.91666667 -0.9125 -0.90833333 -0.90416667 -0.9 -0.89583333 -0.89166667 -0.8875 -0.88333333 -0.87916667 -0.875 -0.87083333 -0.86666667 -0.8625 -0.85833333 -0.85416667 -0.85 -0.84583333 -0.84166667 -0.8375 -0.83333333 -0.82916667 -0.825 -0.82083333 -0.81666667 -0.8125 -0.80833333 -0.80416667 -0.8 -0.79583333 -0.79166667 -0.7875 -0.78333333 -0.77916667 -0.775 -0.77083333 -0.76666667 -0.7625 -0.75833333 -0.75416667 -0.75 -0.74583333 -0.74166667 -0.7375 -0.73333333 -0.72916667 -0.725 -0.72083333 -0.71666667 -0.7125 -0.70833333 -0.70416667 -0.7 -0.69583333 -0.69166667 -0.6875 -0.68333333 -0.67916667 -0.675 -0.67083333 -0.66666667 -0.6625 -0.65833333 -0.65416667 -0.65 -0.64583333 -0.64166667 -0.6375 -0.63333333 -0.62916667 -0.625 -0.62083333 -0.61666667 -0.6125 -0.60833333 -0.60416667 -0.6 -0.59583333 -0.59166667 -0.5875 -0.58333333 -0.57916667 -0.575 -0.57083333 -0.56666667 -0.5625 -0.55833333 -0.55416667 -0.55 -0.54583333 -0.54166667 -0.5375 -0.53333333 -0.52916667 -0.525 -0.52083333 -0.51666667 -0.5125 -0.50833333 -0.50416667 -0.5 -0.49583333 -0.49166667 -0.4875 -0.48333333 -0.47916667 -0.475 -0.47083333 -0.46666667 -0.4625 -0.45833333 -0.45416667 -0.45 -0.44583333 -0.44166667 -0.4375 -0.43333333 -0.42916667 -0.425 -0.42083333 -0.41666667 -0.4125 -0.40833333 -0.40416667 -0.4 -0.39583333 -0.39166667 -0.3875 -0.38333333 -0.37916667 -0.375 -0.37083333 -0.36666667 -0.3625 -0.35833333 -0.35416667 -0.35 -0.34583333 -0.34166667 -0.3375 -0.33333333 -0.32916667 -0.325 -0.32083333 -0.31666667 -0.3125 -0.30833333 -0.30416667 -0.3 -0.29583333 -0.29166667 -0.2875 -0.28333333 -0.27916667 -0.275 -0.27083333 -0.26666667 -0.2625 -0.25833333 -0.25416667 -0.25 -0.24583333 -0.24166667 -0.2375 -0.23333333 -0.22916667 -0.225 -0.22083333 -0.21666667 -0.2125 -0.20833333 -0.20416667 -0.2 -0.19583333 -0.19166667 -0.1875 -0.18333333 -0.17916667 -0.175 -0.17083333 -0.16666667 -0.1625 -0.15833333 -0.15416667 -0.15 -0.14583333 -0.14166667 -0.1375 -0.13333333 -0.12916667 -0.125 -0.12083333 -0.11666667 -0.1125 -0.10833333 -0.10416667 -0.1 -0.09583333 -0.09166667 -0.0875 -0.08333333 -0.07916667 -0.075 -0.07083333 -0.06666667 -0.0625 -0.05833333 -0.05416667 -0.05 -0.04583333 -0.04166667 -0.0375 -0.03333333 -0.02916667 -0.025 -0.02083333 -0.01666667 -0.0125 -0.00833333 -0.00416667 0 0 0 0 0 0
  line L123 (26.8955, 1.5338) -> (26.8948, 1.5341)
  line L124 (26.8948, 1.5341) -> (26.6221, 1.6453)
  arc A58 (26.6221, 1.6453) -> (27.0473, 2.7529) centre (0, 12.5) ccw
  line L125 (27.0473, 2.7529) -> (27.3243, 2.6531)
  line L126 (27.3243, 2.6531) -> (27.3251, 2.6528)
  spline S58 degree 5 poles (27.3251, 2.6528) (27.3252, 2.6528) (27.3254, 2.6527) (27.3257, 2.6526) (27.3262, 2.6525) (27.3269, 2.6522) (27.3277, 2.6519) (27.3286, 2.6516) (27.3296, 2.6513) (27.3308, 2.6509) (27.332, 2.6505) (27.3334, 2.65) (27.3348, 2.6495) (27.3364, 2.649) (27.338, 2.6485) (27.3398, 2.6479) (27.3416, 2.6473) (27.3435, 2.6467) (27.3456, 2.6461) (27.3477, 2.6454) (27.3499, 2.6447) (27.3523, 2.644) (27.3547, 2.6432) (27.3572, 2.6425) (27.3598, 2.6417) (27.3625, 2.6409) (27.3652, 2.64) (27.3681, 2.6392) (27.371, 2.6383) (27.3741, 2.6374) (27.3772, 2.6365) (27.3804, 2.6355) (27.3837, 2.6346) (27.387, 2.6336) (27.3905, 2.6326) (27.394, 2.6316) (27.3976, 2.6306) (27.4013, 2.6296) (27.4051, 2.6285) (27.409, 2.6275) (27.4129, 2.6264) (27.4169, 2.6253) (27.421, 2.6242) (27.4252, 2.6231) (27.4294, 2.622) (27.4337, 2.6208) (27.4381, 2.6197) (27.4426, 2.6185) (27.4471, 2.6173) (27.4517, 2.6162) (27.4564, 2.615) (27.4612, 2.6138) (27.466, 2.6126) (27.4709, 2.6113) (27.4759, 2.6101) (27.481, 2.6089) (27.4861, 2.6076) (27.4912, 2.6064) (27.4965, 2.6051) (27.5018, 2.6038) (27.5072, 2.6026) (27.5127, 2.6013) (27.5182, 2.6) (27.5238, 2.5987) (27.5294, 2.5974) (27.5352, 2.5961) (27.5409, 2.5948) (27.5468, 2.5935) (27.5527, 2.5921) (27.5587, 2.5908) (27.5647, 2.5895) (27.5709, 2.5882) (27.577, 2.5868) (27.5833, 2.5855) (27.5896, 2.5842) (27.5959, 2.5828) (27.6023, 2.5815) (27.6088, 2.5801) (27.6154, 2.5788) (27.622, 2.5775) (27.6286, 2.5761) (27.6353, 2.5748) (27.6421, 2.5734) (27.649, 2.5721) (27.6559, 2.5707) (27.6628, 2.5694) (27.6698, 2.568) (27.6769, 2.5667) (27.6841, 2.5653) (27.6912, 2.564) (27.6985, 2.5626) (27.7058, 2.5613) (27.7132, 2.5599) (27.7206, 2.5586) (27.728, 2.5572) (27.7356, 2.5559) (27.7431, 2.5546) (27.7508, 2.5532) (27.7585, 2.5519) (27.7662, 2.5506) (27.774, 2.5492) (27.7819, 2.5479) (27.7898, 2.5466) (27.7977, 2.5453) (27.8057, 2.544) (27.8138, 2.5427) (27.8219, 2.5414) (27.8301, 2.5401) (27.8383, 2.5388) (27.8466, 2.5375) (27.8549, 2.5362) (27.8633, 2.5349) (27.8717, 2.5336) (27.8802, 2.5324) (27.8887, 2.5311) (27.8973, 2.5299) (27.9059, 2.5286) (27.9146, 2.5274) (27.9233, 2.5261) (27.9321, 2.5249) (27.9409, 2.5237) (27.9498, 2.5224) (27.9587, 2.5212) (27.9677, 2.52) (27.9767, 2.5188) (27.9858, 2.5176) (27.9949, 2.5164) (28.004, 2.5153) (28.0133, 2.5141) (28.0225, 2.5129) (28.0318, 2.5118) (28.0412, 2.5106) (28.0506, 2.5095) (28.06, 2.5084) (28.0695, 2.5072) (28.079, 2.5061) (28.0886, 2.505) (28.0982, 2.5039) (28.1079, 2.5028) (28.1176, 2.5017) (28.1274, 2.5007) (28.1372, 2.4996) (28.147, 2.4986) (28.1569, 2.4975) (28.1668, 2.4965) (28.1768, 2.4955) (28.1868, 2.4945) (28.1969, 2.4935) (28.207, 2.4925) (28.2172, 2.4915) (28.2274, 2.4905) (28.2376, 2.4896) (28.2479, 2.4886) (28.2582, 2.4877) (28.2686, 2.4867) (28.279, 2.4858) (28.2894, 2.4849) (28.2999, 2.484) (28.3105, 2.4831) (28.321, 2.4823) (28.3317, 2.4814) (28.3423, 2.4805) (28.353, 2.4797) (28.3638, 2.4789) (28.3745, 2.4781) (28.3854, 2.4773) (28.3962, 2.4765) (28.4071, 2.4757) (28.4181, 2.4749) (28.429, 2.4742) (28.44, 2.4734) (28.4511, 2.4727) (28.4622, 2.472) (28.4733, 2.4713) (28.4845, 2.4706) (28.4957, 2.4699) (28.507, 2.4692) (28.5183, 2.4686) (28.5296, 2.4679) (28.541, 2.4673) (28.5524, 2.4667) (28.5638, 2.4661) (28.5753, 2.4655) (28.5868, 2.4649) (28.5984, 2.4644) (28.61, 2.4638) (28.6216, 2.4633) (28.6333, 2.4628) (28.645, 2.4623) (28.6567, 2.4618) (28.6685, 2.4613) (28.6803, 2.4608) (28.6922, 2.4604) (28.7041, 2.46) (28.716, 2.4595) (28.728, 2.4591) (28.74, 2.4588) (28.752, 2.4584) (28.7641, 2.458) (28.7762, 2.4577) (28.7883, 2.4573) (28.8005, 2.457) (28.8127, 2.4567) (28.8249, 2.4564) (28.8372, 2.4562) (28.8495, 2.4559) (28.8619, 2.4557) (28.8743, 2.4555) (28.8867, 2.4552) (28.8991, 2.4551) (28.9116, 2.4549) (28.9241, 2.4547) (28.9367, 2.4546) (28.9493, 2.4544) (28.9619, 2.4543) (28.9745, 2.4542) (28.9872, 2.4542) (29, 2.4541) (29.0127, 2.454) (29.0255, 2.454) (29.0383, 2.454) (29.0512, 2.454) (29.0641, 2.454) (29.077, 2.454) (29.0899, 2.4541) (29.1029, 2.4542) (29.1159, 2.4542) (29.129, 2.4543) (29.142, 2.4545) (29.1551, 2.4546) (29.1683, 2.4547) (29.1815, 2.4549) (29.1947, 2.4551) (29.2079, 2.4553) (29.2212, 2.4555) (29.2345, 2.4558) (29.2478, 2.456) (29.2612, 2.4563) (29.2745, 2.4566) (29.288, 2.4569) (29.3014, 2.4572) (29.3122, 2.4575) (29.3203, 2.4577) (29.3257, 2.4578) (29.3284, 2.4579) knots 0 0 0 0 0 0 0.00416667 0.00833333 0.0125 0.01666667 0.02083333 0.025 0.02916667 0.03333333 0.0375 0.04166667 0.04583333 0.05 0.05416667 0.05833333 0.0625 0.06666667 0.07083333 0.075 0.07916667 0.08333333 0.0875 0.09166667 0.09583333 0.1 0.10416667 0.10833333 0.1125 0.11666667 0.12083333 0.125 0.12916667 0.13333333 0.1375 0.14166667 0.14583333 0.15 0.15416667 0.15833333 0.1625 0.16666667 0.17083333 0.175 0.17916667 0.18333333 0.1875 0.19166667 0.19583333 0.2 0.20416667 0.20833333 0.2125 0.21666667 0.22083333 0.225 0.22916667 0.23333333 0.2375 0.24166667 0.24583333 0.25 0.25416667 0.25833333 0.2625 0.26666667 0.27083333 0.275 0.27916667 0.28333333 0.2875 0.29166667 0.29583333 0.3 0.30416667 0.30833333 0.3125 0.31666667 0.32083333 0.325 0.32916667 0.33333333 0.3375 0.34166667 0.34583333 0.35 0.35416667 0.35833333 0.3625 0.36666667 0.37083333 0.375 0.37916667 0.38333333 0.3875 0.39166667 0.39583333 0.4 0.40416667 0.40833333 0.4125 0.41666667 0.42083333 0.425 0.42916667 0.43333333 0.4375 0.44166667 0.44583333 0.45 0.45416667 0.45833333 0.4625 0.46666667 0.47083333 0.475 0.47916667 0.48333333 0.4875 0.49166667 0.49583333 0.5 0.50416667 0.50833333 0.5125 0.51666667 0.52083333 0.525 0.52916667 0.53333333 0.5375 0.54166667 0.54583333 0.55 0.55416667 0.55833333 0.5625 0.56666667 0.57083333 0.575 0.57916667 0.58333333 0.5875 0.59166667 0.59583333 0.6 0.60416667 0.60833333 0.6125 0.61666667 0.62083333 0.625 0.62916667 0.63333333 0.6375 0.64166667 0.64583333 0.65 0.65416667 0.65833333 0.6625 0.66666667 0.67083333 0.675 0.67916667 0.68333333 0.6875 0.69166667 0.69583333 0.7 0.70416667 0.70833333 0.7125 0.71666667 0.72083333 0.725 0.72916667 0.73333333 0.7375 0.74166667 0.74583333 0.75 0.75416667 0.75833333 0.7625 0.76666667 0.77083333 0.775 0.77916667 0.78333333 0.7875 0.79166667 0.79583333 0.8 0.80416667 0.80833333 0.8125 0.81666667 0.82083333 0.825 0.82916667 0.83333333 0.8375 0.84166667 0.84583333 0.85 0.85416667 0.85833333 0.8625 0.86666667 0.87083333 0.875 0.87916667 0.88333333 0.8875 0.89166667 0.89583333 0.9 0.90416667 0.90833333 0.9125 0.91666667 0.92083333 0.925 0.92916667 0.93333333 0.9375 0.94166667 0.94583333 0.95 0.95416667 0.95833333 0.9625 0.96666667 0.97083333 0.975 0.97916667 0.98333333 0.9875 0.99166667 0.99583333 1 1 1 1 1 1
  arc A59 (29.3284, 2.4579) -> (29.6298, 3.3854) centre (0, 12.5) ccw
  spline S59 degree 5 poles (29.6298, 3.3854) (29.6276, 3.3871) (29.6234, 3.3904) (29.6169, 3.3953) (29.6084, 3.4019) (29.5977, 3.41) (29.587, 3.4182) (29.5763, 3.4263) (29.5657, 3.4343) (29.555, 3.4424) (29.5444, 3.4504) (29.5338, 3.4584) (29.5232, 3.4663) (29.5127, 3.4742) (29.5021, 3.4821) (29.4915, 3.4899) (29.481, 3.4978) (29.4705, 3.5055) (29.46, 3.5133) (29.4495, 3.521) (29.4391, 3.5287) (29.4286, 3.5363) (29.4182, 3.544) (29.4078, 3.5515) (29.3974, 3.5591) (29.387, 3.5666) (29.3766, 3.5741) (29.3663, 3.5816) (29.356, 3.589) (29.3457, 3.5964) (29.3354, 3.6037) (29.3251, 3.6111) (29.3148, 3.6184) (29.3046, 3.6256) (29.2944, 3.6329) (29.2842, 3.64) (29.274, 3.6472) (29.2638, 3.6543) (29.2537, 3.6614) (29.2435, 3.6685) (29.2334, 3.6755) (29.2233, 3.6825) (29.2132, 3.6895) (29.2032, 3.6964) (29.1932, 3.7033) (29.1831, 3.7102) (29.1731, 3.717) (29.1632, 3.7238) (29.1532, 3.7306) (29.1433, 3.7374) (29.1334, 3.7441) (29.1235, 3.7507) (29.1136, 3.7574) (29.1037, 3.764) (29.0939, 3.7705) (29.0841, 3.7771) (29.0743, 3.7836) (29.0646, 3.7901) (29.0548, 3.7965) (29.0451, 3.8029) (29.0354, 3.8093) (29.0257, 3.8156) (29.016, 3.8219) (29.0064, 3.8282) (28.9968, 3.8344) (28.9872, 3.8407) (28.9776, 3.8468) (28.9681, 3.853) (28.9586, 3.8591) (28.9491, 3.8652) (28.9396, 3.8712) (28.9302, 3.8772) (28.9207, 3.8832) (28.9113, 3.8891) (28.902, 3.895) (28.8926, 3.9009) (28.8833, 3.9068) (28.874, 3.9126) (28.8647, 3.9183) (28.8555, 3.9241) (28.8462, 3.9298) (28.837, 3.9355) (28.8279, 3.9411) (28.8187, 3.9467) (28.8096, 3.9523) (28.8005, 3.9578) (28.7914, 3.9633) (28.7824, 3.9688) (28.7734, 3.9743) (28.7644, 3.9797) (28.7554, 3.985) (28.7465, 3.9904) (28.7376, 3.9957) (28.7287, 4.001) (28.7199, 4.0062) (28.711, 4.0114) (28.7022, 4.0166) (28.6935, 4.0217) (28.6847, 4.0268) (28.676, 4.0319) (28.6674, 4.037) (28.6587, 4.042) (28.6501, 4.0469) (28.6415, 4.0519) (28.633, 4.0568) (28.6244, 4.0616) (28.616, 4.0665) (28.6075, 4.0713) (28.5991, 4.0761) (28.5907, 4.0808) (28.5823, 4.0855) (28.574, 4.0902) (28.5657, 4.0948) (28.5574, 4.0994) (28.5491, 4.104) (28.5409, 4.1085) (28.5328, 4.113) (28.5246, 4.1175) (28.5165, 4.1219) (28.5085, 4.1263) (28.5004, 4.1307) (28.4924, 4.135) (28.4845, 4.1393) (28.4765, 4.1435) (28.4686, 4.1478) (28.4608, 4.152) (28.4529, 4.1561) (28.4452, 4.1602) (28.4374, 4.1643) (28.4297, 4.1684) (28.422, 4.1724) (28.4144, 4.1764) (28.4068, 4.1804) (28.3992, 4.1843) (28.3917, 4.1882) (28.3842, 4.192) (28.3767, 4.1958) (28.3693, 4.1996) (28.3619, 4.2034) (28.3546, 4.2071) (28.3473, 4.2108) (28.3401, 4.2144) (28.3329, 4.218) (28.3257, 4.2216) (28.3186, 4.2252) (28.3115, 4.2287) (28.3044, 4.2322) (28.2974, 4.2356) (28.2905, 4.239) (28.2835, 4.2424) (28.2767, 4.2457) (28.2698, 4.249) (28.263, 4.2523) (28.2563, 4.2555) (28.2496, 4.2588) (28.2429, 4.2619) (28.2363, 4.2651) (28.2298, 4.2682) (28.2233, 4.2712) (28.2168, 4.2743) (28.2104, 4.2773) (28.204, 4.2802) (28.1977, 4.2831) (28.1914, 4.286) (28.1851, 4.2889) (28.179, 4.2917) (28.1728, 4.2945) (28.1667, 4.2973) (28.1607, 4.3) (28.1547, 4.3027) (28.1488, 4.3053) (28.1429, 4.308) (28.1371, 4.3105) (28.1313, 4.3131) (28.1256, 4.3156) (28.1199, 4.3181) (28.1143, 4.3205) (28.1087, 4.323) (28.1032, 4.3253) (28.0978, 4.3277) (28.0924, 4.33) (28.087, 4.3323) (28.0818, 4.3345) (28.0765, 4.3367) (28.0714, 4.3389) (28.0663, 4.341) (28.0612, 4.3431) (28.0562, 4.3452) (28.0513, 4.3472) (28.0464, 4.3492) (28.0416, 4.3512) (28.0369, 4.3531) (28.0322, 4.355) (28.0276, 4.3568) (28.023, 4.3587) (28.0185, 4.3605) (28.0141, 4.3622) (28.0097, 4.3639) (28.0054, 4.3656) (28.0012, 4.3673) (27.997, 4.3689) (27.9929, 4.3705) (27.9889, 4.372) (27.9849, 4.3735) (27.9811, 4.375) (27.9772, 4.3764) (27.9735, 4.3778) (27.9698, 4.3792) (27.9662, 4.3806) (27.9627, 4.3819) (27.9593, 4.3831) (27.9559, 4.3844) (27.9526, 4.3856) (27.9494, 4.3867) (27.9462, 4.3879) (27.9432, 4.3889) (27.9402, 4.39) (27.9373, 4.391) (27.9345, 4.392) (27.9318, 4.393) (27.9291, 4.3939) (27.9265, 4.3948) (27.9241, 4.3956) (27.9217, 4.3964) (27.9194, 4.3972) (27.9172, 4.398) (27.915, 4.3987) (27.913, 4.3993) (27.9111, 4.4) (27.9092, 4.4006) (27.9075, 4.4012) (27.9058, 4.4017) (27.9043, 4.4022) (27.9028, 4.4027) (27.9015, 4.4031) (27.9002, 4.4035) (27.8991, 4.4038) (27.898, 4.4042) (27.8971, 4.4044) (27.8963, 4.4047) (27.8956, 4.4049) (27.8951, 4.4051) (27.8948, 4.4052) (27.8946, 4.4052) (27.8945, 4.4052) knots -1 -1 -1 -1 -1 -1 -0.99583333 -0.99166667 -0.9875 -0.98333333 -0.97916667 -0.975 -0.97083333 -0.96666667 -0.9625 -0.95833333 -0.95416667 -0.95 -0.94583333 -0.94166667 -0.9375 -0.93333333 -0.92916667 -0.925 -0.92083333 -0.91666667 -0.9125 -0.90833333 -0.90416667 -0.9 -0.89583333 -0.89166667 -0.8875 -0.88333333 -0.87916667 -0.875 -0.87083333 -0.86666667 -0.8625 -0.85833333 -0.85416667 -0.85 -0.84583333 -0.84166667 -0.8375 -0.83333333 -0.82916667 -0.825 -0.82083333 -0.81666667 -0.8125 -0.80833333 -0.80416667 -0.8 -0.79583333 -0.79166667 -0.7875 -0.78333333 -0.77916667 -0.775 -0.77083333 -0.76666667 -0.7625 -0.75833333 -0.75416667 -0.75 -0.74583333 -0.74166667 -0.7375 -0.73333333 -0.72916667 -0.725 -0.72083333 -0.71666667 -0.7125 -0.70833333 -0.70416667 -0.7 -0.69583333 -0.69166667 -0.6875 -0.68333333 -0.67916667 -0.675 -0.67083333 -0.66666667 -0.6625 -0.65833333 -0.65416667 -0.65 -0.64583333 -0.64166667 -0.6375 -0.63333333 -0.62916667 -0.625 -0.62083333 -0.61666667 -0.6125 -0.60833333 -0.60416667 -0.6 -0.59583333 -0.59166667 -0.5875 -0.58333333 -0.57916667 -0.575 -0.57083333 -0.56666667 -0.5625 -0.55833333 -0.55416667 -0.55 -0.54583333 -0.54166667 -0.5375 -0.53333333 -0.52916667 -0.525 -0.52083333 -0.51666667 -0.5125 -0.50833333 -0.50416667 -0.5 -0.49583333 -0.49166667 -0.4875 -0.48333333 -0.47916667 -0.475 -0.47083333 -0.46666667 -0.4625 -0.45833333 -0.45416667 -0.45 -0.44583333 -0.44166667 -0.4375 -0.43333333 -0.42916667 -0.425 -0.42083333 -0.41666667 -0.4125 -0.40833333 -0.40416667 -0.4 -0.39583333 -0.39166667 -0.3875 -0.38333333 -0.37916667 -0.375 -0.37083333 -0.36666667 -0.3625 -0.35833333 -0.35416667 -0.35 -0.34583333 -0.34166667 -0.3375 -0.33333333 -0.32916667 -0.325 -0.32083333 -0.31666667 -0.3125 -0.30833333 -0.30416667 -0.3 -0.29583333 -0.29166667 -0.2875 -0.28333333 -0.27916667 -0.275 -0.27083333 -0.26666667 -0.2625 -0.25833333 -0.25416667 -0.25 -0.24583333 -0.24166667 -0.2375 -0.23333333 -0.22916667 -0.225 -0.22083333 -0.21666667 -0.2125 -0.20833333 -0.20416667 -0.2 -0.19583333 -0.19166667 -0.1875 -0.18333333 -0.17916667 -0.175 -0.17083333 -0.16666667 -0.1625 -0.15833333 -0.15416667 -0.15 -0.14583333 -0.14166667 -0.1375 -0.13333333 -0.12916667 -0.125 -0.12083333 -0.11666667 -0.1125 -0.10833333 -0.10416667 -0.1 -0.09583333 -0.09166667 -0.0875 -0.08333333 -0.07916667 -0.075 -0.07083333 -0.06666667 -0.0625 -0.05833333 -0.05416667 -0.05 -0.04583333 -0.04166667 -0.0375 -0.03333333 -0.02916667 -0.025 -0.02083333 -0.01666667 -0.0125 -0.00833333 -0.00416667 0 0 0 0 0 0
  line L127 (27.8945, 4.4052) -> (27.8937, 4.4055)
  line L128 (27.8937, 4.4055) -> (27.6109, 4.4875)
  arc A60 (27.6109, 4.4875) -> (27.918, 5.6335) centre (0, 12.5) ccw
  line L129 (27.918, 5.6335) -> (28.2039, 5.5632)
  line L130 (28.2039, 5.5632) -> (28.2047, 5.563)
  spline S60 degree 5 poles (28.2047, 5.563) (28.2048, 5.563) (28.205, 5.563) (28.2053, 5.5629) (28.2058, 5.5628) (28.2065, 5.5626) (28.2074, 5.5624) (28.2083, 5.5622) (28.2094, 5.5619) (28.2106, 5.5617) (28.2118, 5.5614) (28.2132, 5.5611) (28.2147, 5.5608) (28.2163, 5.5604) (28.218, 5.5601) (28.2198, 5.5597) (28.2217, 5.5593) (28.2237, 5.5589) (28.2258, 5.5584) (28.228, 5.558) (28.2303, 5.5575) (28.2327, 5.5571) (28.2351, 5.5566) (28.2377, 5.5561) (28.2404, 5.5555) (28.2431, 5.555) (28.246, 5.5545) (28.2489, 5.5539) (28.2519, 5.5534) (28.255, 5.5528) (28.2582, 5.5522) (28.2615, 5.5516) (28.2649, 5.551) (28.2683, 5.5504) (28.2719, 5.5498) (28.2755, 5.5492) (28.2792, 5.5485) (28.283, 5.5479) (28.2868, 5.5472) (28.2908, 5.5466) (28.2948, 5.5459) (28.2989, 5.5453) (28.3031, 5.5446) (28.3074, 5.5439) (28.3117, 5.5432) (28.3161, 5.5426) (28.3206, 5.5419) (28.3252, 5.5412) (28.3298, 5.5405) (28.3345, 5.5398) (28.3393, 5.5391) (28.3442, 5.5384) (28.3491, 5.5377) (28.3541, 5.537) (28.3592, 5.5363) (28.3643, 5.5356) (28.3695, 5.5349) (28.3748, 5.5342) (28.3802, 5.5335) (28.3856, 5.5328) (28.3911, 5.5321) (28.3966, 5.5314) (28.4023, 5.5307) (28.408, 5.53) (28.4137, 5.5293) (28.4196, 5.5286) (28.4255, 5.5279) (28.4314, 5.5272) (28.4374, 5.5265) (28.4435, 5.5258) (28.4497, 5.5251) (28.4559, 5.5244) (28.4622, 5.5237) (28.4685, 5.5231) (28.4749, 5.5224) (28.4814, 5.5217) (28.4879, 5.5211) (28.4945, 5.5204) (28.5011, 5.5197) (28.5078, 5.5191) (28.5146, 5.5184) (28.5214, 5.5178) (28.5283, 5.5172) (28.5353, 5.5165) (28.5423, 5.5159) (28.5493, 5.5153) (28.5564, 5.5147) (28.5636, 5.5141) (28.5709, 5.5135) (28.5781, 5.5129) (28.5855, 5.5123) (28.5929, 5.5118) (28.6004, 5.5112) (28.6079, 5.5106) (28.6154, 5.5101) (28.6231, 5.5095) (28.6307, 5.509) (28.6385, 5.5085) (28.6463, 5.5079) (28.6541, 5.5074) (28.662, 5.5069) (28.67, 5.5064) (28.678, 5.506) (28.686, 5.5055) (28.6941, 5.505) (28.7023, 5.5046) (28.7105, 5.5041) (28.7187, 5.5037) (28.727, 5.5032) (28.7354, 5.5028) (28.7438, 5.5024) (28.7523, 5.502) (28.7608, 5.5016) (28.7694, 5.5013) (28.778, 5.5009) (28.7866, 5.5005) (28.7953, 5.5002) (28.8041, 5.4999) (28.8129, 5.4995) (28.8218, 5.4992) (28.8307, 5.4989) (28.8396, 5.4986) (28.8486, 5.4984) (28.8577, 5.4981) (28.8668, 5.4979) (28.8759, 5.4976) (28.8851, 5.4974) (28.8943, 5.4972) (28.9036, 5.497) (28.9129, 5.4968) (28.9223, 5.4966) (28.9317, 5.4964) (28.9412, 5.4963) (28.9507, 5.4962) (28.9602, 5.496) (28.9698, 5.4959) (28.9795, 5.4958) (28.9892, 5.4957) (28.9989, 5.4957) (29.0087, 5.4956) (29.0185, 5.4956) (29.0284, 5.4955) (29.0383, 5.4955) (29.0482, 5.4955) (29.0582, 5.4955) (29.0682, 5.4956) (29.0783, 5.4956) (29.0884, 5.4957) (29.0986, 5.4957) (29.1088, 5.4958) (29.119, 5.4959) (29.1293, 5.496) (29.1396, 5.4962) (29.15, 5.4963) (29.1604, 5.4965) (29.1708, 5.4966) (29.1813, 5.4968) (29.1919, 5.497) (29.2024, 5.4972) (29.213, 5.4975) (29.2237, 5.4977) (29.2344, 5.498) (29.2451, 5.4983) (29.2559, 5.4986) (29.2667, 5.4989) (29.2775, 5.4992) (29.2884, 5.4996) (29.2993, 5.4999) (29.3103, 5.5003) (29.3213, 5.5007) (29.3323, 5.5011) (29.3434, 5.5016) (29.3545, 5.502) (29.3657, 5.5025) (29.3768, 5.503) (29.3881, 5.5035) (29.3993, 5.504) (29.4106, 5.5045) (29.422, 5.505) (29.4333, 5.5056) (29.4447, 5.5062) (29.4562, 5.5068) (29.4677, 5.5074) (29.4792, 5.508) (29.4907, 5.5087) (29.5023, 5.5094) (29.514, 5.51) (29.5256, 5.5108) (29.5373, 5.5115) (29.549, 5.5122) (29.5608, 5.513) (29.5726, 5.5137) (29.5844, 5.5145) (29.5963, 5.5154) (29.6082, 5.5162) (29.6201, 5.517) (29.6321, 5.5179) (29.6441, 5.5188) (29.6562, 5.5197) (29.6682, 5.5206) (29.6803, 5.5216) (29.6925, 5.5225) (29.7047, 5.5235) (29.7169, 5.5245) (29.7291, 5.5255) (29.7414, 5.5265) (29.7537, 5.5276) (29.766, 5.5287) (29.7784, 5.5298) (29.7908, 5.5309) (29.8032, 5.532) (29.8157, 5.5331) (29.8282, 5.5343) (29.8407, 5.5355) (29.8533, 5.5367) (29.8659, 5.5379) (29.8785, 5.5392) (29.8912, 5.5404) (29.9039, 5.5417) (29.9166, 5.543) (29.9293, 5.5444) (29.9421, 5.5457) (29.9549, 5.5471) (29.9678, 5.5484) (29.9806, 5.5499) (29.9935, 5.5513) (30.0065, 5.5527) (30.0194, 5.5542) (30.0324, 5.5557) (30.0455, 5.5572) (30.0585, 5.5587) (30.0716, 5.5602) (30.0847, 5.5618) (30.0979, 5.5634) (30.111, 5.565) (30.1242, 5.5666) (30.1375, 5.5683) (30.1507, 5.5699) (30.164, 5.5716) (30.1773, 5.5733) (30.1907, 5.575) (30.2014, 5.5764) (30.2094, 5.5775) (30.2148, 5.5782) (30.2174, 5.5786) knots 0 0 0 0 0 0 0.00416667 0.00833333 0.0125 0.01666667 0.02083333 0.025 0.02916667 0.03333333 0.0375 0.04166667 0.04583333 0.05 0.05416667 0.05833333 0.0625 0.06666667 0.07083333 0.075 0.07916667 0.08333333 0.0875 0.09166667 0.09583333 0.1 0.10416667 0.10833333 0.1125 0.11666667 0.12083333 0.125 0.12916667 0.13333333 0.1375 0.14166667 0.14583333 0.15 0.15416667 0.15833333 0.1625 0.16666667 0.17083333 0.175 0.17916667 0.18333333 0.1875 0.19166667 0.19583333 0.2 0.20416667 0.20833333 0.2125 0.21666667 0.22083333 0.225 0.22916667 0.23333333 0.2375 0.24166667 0.24583333 0.25 0.25416667 0.25833333 0.2625 0.26666667 0.27083333 0.275 0.27916667 0.28333333 0.2875 0.29166667 0.29583333 0.3 0.30416667 0.30833333 0.3125 0.31666667 0.32083333 0.325 0.32916667 0.33333333 0.3375 0.34166667 0.34583333 0.35 0.35416667 0.35833333 0.3625 0.36666667 0.37083333 0.375 0.37916667 0.38333333 0.3875 0.39166667 0.39583333 0.4 0.40416667 0.40833333 0.4125 0.41666667 0.42083333 0.425 0.42916667 0.43333333 0.4375 0.44166667 0.44583333 0.45 0.45416667 0.45833333 0.4625 0.46666667 0.47083333 0.475 0.47916667 0.48333333 0.4875 0.49166667 0.49583333 0.5 0.50416667 0.50833333 0.5125 0.51666667 0.52083333 0.525 0.52916667 0.53333333 0.5375 0.54166667 0.54583333 0.55 0.55416667 0.55833333 0.5625 0.56666667 0.57083333 0.575 0.57916667 0.58333333 0.5875 0.59166667 0.59583333 0.6 0.60416667 0.60833333 0.6125 0.61666667 0.62083333 0.625 0.62916667 0.63333333 0.6375 0.64166667 0.64583333 0.65 0.65416667 0.65833333 0.6625 0.66666667 0.67083333 0.675 0.67916667 0.68333333 0.6875 0.69166667 0.69583333 0.7 0.70416667 0.70833333 0.7125 0.71666667 0.72083333 0.725 0.72916667 0.73333333 0.7375 0.74166667 0.74583333 0.75 0.75416667 0.75833333 0.7625 0.76666667 0.77083333 0.775 0.77916667 0.78333333 0.7875 0.79166667 0.79583333 0.8 0.80416667 0.80833333 0.8125 0.81666667 0.82083333 0.825 0.82916667 0.83333333 0.8375 0.84166667 0.84583333 0.85 0.85416667 0.85833333 0.8625 0.86666667 0.87083333 0.875 0.87916667 0.88333333 0.8875 0.89166667 0.89583333 0.9 0.90416667 0.90833333 0.9125 0.91666667 0.92083333 0.925 0.92916667 0.93333333 0.9375 0.94166667 0.94583333 0.95 0.95416667 0.95833333 0.9625 0.96666667 0.97083333 0.975 0.97916667 0.98333333 0.9875 0.99166667 0.99583333 1 1 1 1 1 1
  arc A61 (30.2174, 5.5786) -> (30.4202, 6.5325) centre (0, 12.5) ccw